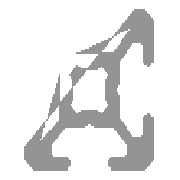
# Autodesk Inventor part: 3 842 992 890-25mm
Saved by Autodesk Inventor 2011 SP1 (Build 150282100, 282)
## iProperties
Created: 2011-02-24
Part Number: 3 842 992 890-25mm
Description: PROFILE 20x20R, -/-
Document SubType Name: Modeling
Designer: SRW
Density: 2.71 g/cm^3
Categories: <MemberInstance><Categories><Category DisplayName="Structural Shapes" InternalName="089c4875-fa83-4c05-b084-43b9cc11f5ed" Mnemonic="GRDR"><CategoryParameter DisplayName="Custom Base Point" InternalName="4f1d1b73-316d-484b-a3df-9cbabb16eb77" Mnemonic="shpBasePoint"/><CategoryParameter DisplayName="FG Authored" InternalName="9c666724-f362-4ea7-ac62-f6a007de5c69" Mnemonic="shpFGAuto"/><CategoryParameter DisplayName="Legacy Member ID" InternalName="340afe4f-75d7-48d3-ab7d-943f3c3da468" Mnemonic="LegacyMemberID"/><CategoryParameter DisplayName="Base Length" InternalName="42e34263-8f20-4d0e-ad48-bf1385b87c24" Mnemonic="shplen"/><CategoryParameter DisplayName="Distance of the Center of Gravity X-X" InternalName="26c9bdb8-9c79-4b4f-a92e-8e197583c9c4" Mnemonic="grcendistX"/><CategoryParameter DisplayName="Distance of the Center of Gravity Y-Y" InternalName="bcc4fb17-7af4-436a-8f8c-d0aa3b0248c5" Mnemonic="grcendistY"/><CategoryParameter DisplayName="Torsional Rigidity Modulus" InternalName="26c1ec35-5026-4c63-ad0a-751cf684a536" Mnemonic="torrigmod"/><CategoryParameter DisplayName="Torsional Section Modulus" InternalName="7c55a8dc-8844-49f9-a867-cc677b30ec9a" Mnemonic="torsecmod"/><CategoryParameter DisplayName="Coefficient of Shear Displacement" InternalName="de4c90c6-aaa8-468f-a335-6737b311b5d3" Mnemonic="shdispc"/><CategoryParameter DisplayName="Section Area" InternalName="1ff91680-64b0-4202-b9a3-7fd3f94bba3b" Mnemonic="secarea"/><CategoryParameter DisplayName="Moment of Inertia (x)" InternalName="4cd780bc-73d7-43ac-917a-579e5cbd684d" Mnemonic="inermomx"/><CategoryParameter DisplayName="Moment of Inertia (y)" InternalName="4b9f58ea-bced-460e-81ea-3d29ca5a49e3" Mnemonic="inermomy"/><CategoryParameter DisplayName="Section Module (x)" InternalName="72cfad18-cf51-4ed4-aaa7-c6b224f8419f" Mnemonic="secmodx"/><CategoryParameter DisplayName="Section Module (y)" InternalName="59eaa5e9-d227-48dc-b6c1-6920f96e0f95" Mnemonic="secmody"/><CategoryParameter DisplayName="Radius of Gyration (x)" InternalName="25778675-03e9-40c1-b6a8-4a9ed693320d" Mnemonic="gyrradx"/><CategoryParameter DisplayName="Radius of Gyration (y)" InternalName="bfa18ebe-1636-4dbe-8d42-b263e0b73184" Mnemonic="gyrrady"/><CategoryParameter DisplayName="Shape Thickness" InternalName="d109cf76-8eb4-42fc-9800-4409734adc67" Mnemonic="shpthick"/><CategoryParameter DisplayName="Second Shape Thickness" InternalName="9251a8e1-85fd-4e47-af99-afdb762317d9" Mnemonic="shpthick2"/><CategoryParameter DisplayName="Shape Width" InternalName="7c717d54-a18f-4666-b4d4-573cce22c62c" Mnemonic="shpwdth"/><CategoryParameter DisplayName="Shape Height" InternalName="50274e7d-5ac0-4796-92cb-c59e54983c67" Mnemonic="shpheig"/><CategoryParameter DisplayName="Mass per Length Unit" InternalName="0bb95a10-148f-4027-a459-38d7b056702a" Mnemonic="shpmass"/><CategoryParameter DisplayName="Section Designation" InternalName="5a64d034-428d-49c8-ba32-7619764de20f" Mnemonic="shpdes"/><Category DisplayName="Other" InternalName="f02205ff-2390-476f-921c-0b3185f88e84" Mnemonic="OTHSHP"><CategoryParameter DisplayName="Moment of Inertia (x)" InternalName="ec6737bc-264f-43ed-b0bd-f6d410c2718d" Mnemonic="inermomx"/><CategoryParameter DisplayName="Moment of Inertia (y)" InternalName="044c654e-f649-48ac-84cc-650a29ae31ca" Mnemonic="inermomy"/><CategoryParameter DisplayName="Section Module (x)" InternalName="cac70804-9d39-43bb-be17-56ea1f39a6c2" Mnemonic="secmodx"/><CategoryParameter DisplayName="Section Module (y)" InternalName="88b8bff9-a616-4028-93d5-ed4f79680d13" Mnemonic="secmody"/><CategoryParameter DisplayName="Section Area" InternalName="c46ecdf8-b6eb-4db9-8b25-30258930c1e3" Mnemonic="secarea"/><CategoryParameter DisplayName="Radius of Gyration (x)" InternalName="ee72c61e-565e-4fd6-b448-66e1e1abcb7e" Mnemonic="gyrradx"/><CategoryParameter DisplayName="Radius of Gyration (y)" InternalName="743e1dfe-1bba-408b-b985-cf752b207386" Mnemonic="gyrrady"/><CategoryParameter DisplayName="Shape Thickness" InternalName="12b1a788-9233-48fd-a933-2df8ff42b15f" Mnemonic="shpthick"/><CategoryParameter DisplayName="Mass per Length Unit" InternalName="2fd289d6-9394-4d2d-97e6-6659d7d4551d" Mnemonic="shpmass"/></Category></Category></Categories><FamilyTemplate Id="20x20R"><FamilyTemplateParameters><FamilyTemplateParameter ObjectType="kUserParameterObject" ValueType="xs:double" Id="1" ObjectReferenceKey="G_L"/><FamilyTemplateParameter ObjectType="kUserParameterObject" ValueType="xs:double" Id="2" ObjectReferenceKey="G_OFFSET_END"/><FamilyTemplateParameter ObjectType="kUserParameterObject" ValueType="xs:double" Id="3" ObjectReferenceKey="G_OFFSET_START"/><FamilyTemplateParameter ObjectType="kUserParameterObject" ValueType="xs:double" Id="4" ObjectReferenceKey="Length"/><FamilyTemplateParameter ObjectType="kPropertyObject" ValueType="xs:string" Id="7" ObjectReferenceKey="{32853F0F-3444-11d1-9E93-0060B03C1CA6}" SubObjectId="52"/><FamilyTemplateParameter ObjectType="kPartComponentDefinitionObject" ValueType="xs:string" Id="8" SubObjectId="Material"/><FamilyTemplateParameter ObjectType="kPropertyObject" ValueType="xs:string" Id="9" ObjectReferenceKey="{32853F0F-3444-11d1-9E93-0060B03C1CA6}" SubObjectId="5"/><FamilyTemplateParameter ObjectType="kPropertyObject" ValueType="xs:string" Id="10" ObjectReferenceKey="{32853F0F-3444-11D1-9E93-0060B03C1CA6}" SubObjectId="55"/><FamilyTemplateParameter ObjectType="kiPartTableColumnObject" ValueType="xs:string" Id="19" ObjectReferenceKey="FILENAME"/><FamilyTemplateParameter ObjectType="kiPartTableColumnObject" ValueType="xs:string" Id="20" ObjectReferenceKey="MEMBER_REVISION"/></FamilyTemplateParameters></FamilyTemplate><CategoryParameterMap><ParamToTemplateMap><ParamToTemplate CategoryParameter="//CategoryParameter[@InternalName='2675968c-4ce5-49e0-a4f5-552d29089031']" TemplateParameter="7"/><ParamToTemplate CategoryParameter="//CategoryParameter[@InternalName='8b46a4cc-9585-4fed-90c3-899f57e09a73']" TemplateParameter="19"/><ParamToTemplate CategoryParameter="//CategoryParameter[@InternalName='42e34263-8f20-4d0e-ad48-bf1385b87c24']" TemplateParameter="4"/><ParamToTemplate CategoryParameter="//CategoryParameter[@InternalName='818a152a-d3c3-49ca-80ee-df7d91421b8e']" TemplateParameter="8"/><ParamToTemplate CategoryParameter="//CategoryParameter[@InternalName='a65d44b9-392f-4f4f-857b-e4b3d54996fe']" TemplateParameter="20"/><ParamToTemplate CategoryParameter="//CategoryParameter[@InternalName='016b6077-bfbe-49bd-92c9-d8d59c39c941']" TemplateParameter="9"/><ParamToTemplate CategoryParameter="//CategoryParameter[@InternalName='9c666724-f362-4ea7-ac62-f6a007de5c69']" ConstantValue="1"/></ParamToTemplateMap></CategoryParameterMap></MemberInstance>
Stock Number: 3 842 992 890
Material: Aluminum-6061
Mass: 11.0537 g
Surface Area: 46.8226 cm^2
Volume: 4.07885 cm^3
Author: SRW
Autodesk Inventor part; units mm, degrees
ref_plane "YZ Plane" through (0, 0, 0) normal (1, 0, 0) x (0, 1, 0)
ref_plane "XZ Plane" through (0, 0, 0) normal (0, 1, 0) x (-1, 0, 0)
ref_plane "XY Plane" through (0, 0, 0) normal (0, 0, 1) x (1, 0, 0)
sketch "20x20R" plane through (0, 0, 0) normal (0, 0, 1) x (1, 0, 0)
  line L0 (187.9019, 38.2996) -> (189.9183, 38.2996)
  arc A0 (187.9019, 38.2996) -> (187.4101, 37.8078) centre (187.9019, 37.8078) ccw
  line L1 (187.4101, 37.0755) -> (187.4101, 37.8078)
  arc A1 (187.4101, 37.0755) -> (187.566, 36.7127) centre (187.9101, 37.0755) ccw
  line L2 (189.8338, 34.5619) -> (187.566, 36.7127)
  arc A2 (189.8338, 34.5619) -> (190.1778, 34.4247) centre (190.1778, 34.9247) ccw
  line L3 (192.4565, 34.4247) -> (190.1778, 34.4247)
  arc A3 (192.5565, 34.3979) -> (192.4565, 34.4247) centre (192.4565, 34.2247) ccw
  line L4 (193.3101, 33.9628) -> (192.5565, 34.3979)
  arc A4 (193.3101, 33.9628) -> (193.5101, 33.9628) centre (193.4101, 34.1361) ccw
  line L5 (194.2637, 34.3979) -> (193.5101, 33.9628)
  arc A5 (194.3637, 34.4247) -> (194.2637, 34.3979) centre (194.3637, 34.2247) ccw
  line L6 (196.6423, 34.4247) -> (194.3637, 34.4247)
  arc A6 (196.6423, 34.4247) -> (196.9864, 34.5619) centre (196.6423, 34.9247) ccw
  arc A7 (191.4101, 25.3593) -> (191.1101, 24.4593) centre (191.4101, 24.8593) ccw
  arc A8 (191.1101, 24.4593) -> (199.5953, 21.3807) centre (200.4101, 36.8593) ccw
  arc A9 (199.5953, 21.3807) -> (199.9751, 22.2336) centre (199.6216, 21.88) ccw
  line L7 (199.9751, 22.2336) -> (196.9959, 25.2128)
  arc A10 (196.9959, 25.2128) -> (196.6423, 25.3593) centre (196.6423, 24.8593) ccw
  line L8 (196.6423, 25.3593) -> (191.4101, 25.3593)
  line L9 (188.9101, 27.8593) -> (188.9101, 33.0915)
  arc A11 (188.9101, 33.0915) -> (188.7636, 33.4451) centre (188.4101, 33.0915) ccw
  line L10 (188.7636, 33.4451) -> (185.7844, 36.4243)
  arc A12 (185.7844, 36.4243) -> (184.9315, 36.0445) centre (185.4308, 36.0708) ccw
  arc A13 (184.9315, 36.0445) -> (188.0101, 27.5593) centre (200.4101, 36.8593) ccw
  arc A14 (188.0101, 27.5593) -> (188.9101, 27.8593) centre (188.4101, 27.8593) ccw
  arc A15 (194.6683, 32.3046) -> (192.1519, 32.3046) centre (193.4101, 29.8593) ccw
  line L11 (192.1519, 32.3046) -> (191.523, 32.807)
  arc A16 (191.523, 32.807) -> (190.4624, 31.7463) centre (193.4101, 29.8593) ccw
  line L12 (190.4624, 31.7463) -> (190.9648, 31.1175)
  arc A17 (190.9648, 31.1175) -> (190.9648, 28.6011) centre (193.4101, 29.8593) ccw
  line L13 (190.9648, 28.6011) -> (190.4624, 27.9722)
  arc A18 (190.4624, 27.9722) -> (191.523, 26.9116) centre (193.4101, 29.8593) ccw
  line L14 (191.523, 26.9116) -> (192.1519, 27.414)
  arc A19 (192.1519, 27.414) -> (194.6683, 27.414) centre (193.4101, 29.8593) ccw
  line L15 (194.6683, 27.414) -> (195.2971, 26.9116)
  arc A20 (195.2971, 26.9116) -> (196.3578, 27.9722) centre (193.4101, 29.8593) ccw
  line L16 (196.3578, 27.9722) -> (195.8554, 28.6011)
  arc A21 (195.8554, 28.6011) -> (195.8554, 31.1175) centre (193.4101, 29.8593) ccw
  line L17 (195.8554, 31.1175) -> (196.3578, 31.7463)
  arc A22 (196.3578, 31.7463) -> (195.2971, 32.807) centre (193.4101, 29.8593) ccw
  line L18 (195.2971, 32.807) -> (194.6683, 32.3046)
  line L19 (199.2541, 36.7127) -> (196.9864, 34.5619)
  arc A23 (199.2541, 36.7127) -> (199.4101, 37.0755) centre (198.9101, 37.0755) ccw
  line L20 (199.4101, 37.8078) -> (199.4101, 37.0755)
  arc A24 (199.4101, 37.8078) -> (198.9183, 38.2996) centre (198.9183, 37.8078) ccw
  line L21 (196.9019, 38.2996) -> (198.9183, 38.2996)
  arc A25 (196.4101, 38.7914) -> (196.9019, 38.2996) centre (196.9019, 38.7914) ccw
  line L22 (196.4101, 39.1093) -> (196.4101, 38.7914)
  arc A26 (196.6101, 39.3093) -> (196.4101, 39.1093) centre (196.6101, 39.1093) ccw
  line L23 (196.7601, 39.3093) -> (196.6101, 39.3093)
  arc A27 (196.7601, 39.3093) -> (196.9601, 39.5093) centre (196.7601, 39.5093) ccw
  line L24 (196.9601, 39.6593) -> (196.9601, 39.5093)
  arc A28 (197.1601, 39.8593) -> (196.9601, 39.6593) centre (197.1601, 39.6593) ccw
  line L25 (201.9101, 39.8593) -> (197.1601, 39.8593)
  arc A29 (203.4101, 38.3593) -> (201.9101, 39.8593) centre (201.9101, 38.3593) ccw
  line L26 (203.4101, 33.6093) -> (203.4101, 38.3593)
  arc A30 (203.2101, 33.4093) -> (203.4101, 33.6093) centre (203.2101, 33.6093) ccw
  line L27 (203.0601, 33.4093) -> (203.2101, 33.4093)
  arc A31 (203.0601, 33.4093) -> (202.8601, 33.2093) centre (203.0601, 33.2093) ccw
  line L28 (202.8601, 33.0593) -> (202.8601, 33.2093)
  arc A32 (202.6601, 32.8593) -> (202.8601, 33.0593) centre (202.6601, 33.0593) ccw
  line L29 (202.2767, 32.8593) -> (202.6601, 32.8593)
  arc A33 (201.7849, 33.3511) -> (202.2767, 32.8593) centre (202.2767, 33.3511) ccw
  line L30 (201.7849, 35.3675) -> (201.7849, 33.3511)
  arc A34 (201.7849, 35.3675) -> (201.2931, 35.8593) centre (201.2931, 35.3675) ccw
  line L31 (200.5609, 35.8593) -> (201.2931, 35.8593)
  arc A35 (200.5609, 35.8593) -> (200.1981, 35.7034) centre (200.5609, 35.3593) ccw
  line L32 (198.0473, 33.4356) -> (200.1981, 35.7034)
  arc A36 (198.0473, 33.4356) -> (197.9101, 33.0915) centre (198.4101, 33.0915) ccw
  line L33 (197.9101, 30.8129) -> (197.9101, 33.0915)
  arc A37 (197.8833, 30.7129) -> (197.9101, 30.8129) centre (197.7101, 30.8129) ccw
  line L34 (197.4482, 29.9593) -> (197.8833, 30.7129)
  arc A38 (197.4482, 29.9593) -> (197.4482, 29.7593) centre (197.6214, 29.8593) ccw
  line L35 (197.8833, 29.0057) -> (197.4482, 29.7593)
  arc A39 (197.9101, 28.9057) -> (197.8833, 29.0057) centre (197.7101, 28.9057) ccw
  line L36 (197.9101, 26.627) -> (197.9101, 28.9057)
  arc A40 (197.9101, 26.627) -> (198.0473, 26.283) centre (198.4101, 26.627) ccw
  line L37 (200.1981, 24.0152) -> (198.0473, 26.283)
  arc A41 (200.1981, 24.0152) -> (200.5609, 23.8593) centre (200.5609, 24.3593) ccw
  line L38 (201.2931, 23.8593) -> (200.5609, 23.8593)
  arc A42 (201.2931, 23.8593) -> (201.7849, 24.3511) centre (201.2931, 24.3511) ccw
  line L39 (201.7849, 26.3675) -> (201.7849, 24.3511)
  arc A43 (202.2767, 26.8593) -> (201.7849, 26.3675) centre (202.2767, 26.3675) ccw
  line L40 (202.6601, 26.8593) -> (202.2767, 26.8593)
  arc A44 (202.8601, 26.6593) -> (202.6601, 26.8593) centre (202.6601, 26.6593) ccw
  line L41 (202.8601, 26.5093) -> (202.8601, 26.6593)
  arc A45 (202.8601, 26.5093) -> (203.0601, 26.3093) centre (203.0601, 26.5093) ccw
  line L42 (203.2101, 26.3093) -> (203.0601, 26.3093)
  arc A46 (203.4101, 26.1093) -> (203.2101, 26.3093) centre (203.2101, 26.1093) ccw
  line L43 (203.4101, 21.3593) -> (203.4101, 26.1093)
  arc A47 (201.9101, 19.8593) -> (203.4101, 21.3593) centre (201.9101, 21.3593) ccw
  line L44 (200.4101, 19.8593) -> (201.9101, 19.8593)
  arc A48 (183.4101, 36.8593) -> (200.4101, 19.8593) centre (200.4101, 36.8593) ccw
  line L45 (183.4101, 38.3593) -> (183.4101, 36.8593)
  arc A49 (184.9101, 39.8593) -> (183.4101, 38.3593) centre (184.9101, 38.3593) ccw
  line L46 (189.6601, 39.8593) -> (184.9101, 39.8593)
  arc A50 (189.8601, 39.6593) -> (189.6601, 39.8593) centre (189.6601, 39.6593) ccw
  line L47 (189.8601, 39.5093) -> (189.8601, 39.6593)
  arc A51 (189.8601, 39.5093) -> (190.0601, 39.3093) centre (190.0601, 39.5093) ccw
  line L48 (190.2101, 39.3093) -> (190.0601, 39.3093)
  arc A52 (190.4101, 39.1093) -> (190.2101, 39.3093) centre (190.2101, 39.1093) ccw
  line L49 (190.4101, 38.7914) -> (190.4101, 39.1093)
  arc A53 (189.9183, 38.2996) -> (190.4101, 38.7914) centre (189.9183, 38.7914) ccw
sketch "Sketch1" plane through (0, 0, 0) normal (0, 0, 1) x (1, 0, 0)
  line L0 (8.4403, 5.5082) -> (8.4403, 3.4918)
  arc A0 (8.4403, 5.5082) -> (7.9485, 6) centre (7.9485, 5.5082) ccw
  line L1 (7.2162, 6) -> (7.9485, 6)
  arc A1 (7.2162, 6) -> (6.8535, 5.8441) centre (7.2162, 5.5) ccw
  line L2 (4.7027, 3.5763) -> (6.8535, 5.8441)
  arc A2 (4.7027, 3.5763) -> (4.5654, 3.2322) centre (5.0654, 3.2322) ccw
  line L3 (4.5654, 0.9536) -> (4.5654, 3.2322)
  arc A3 (4.5387, 0.8536) -> (4.5654, 0.9536) centre (4.3654, 0.9536) ccw
  line L4 (4.1036, 0.1) -> (4.5387, 0.8536)
  arc A4 (4.1036, 0.1) -> (4.1036, -0.1) centre (4.2768, 0) ccw
  line L5 (4.5387, -0.8536) -> (4.1036, -0.1)
  arc A5 (4.5654, -0.9536) -> (4.5387, -0.8536) centre (4.3654, -0.9536) ccw
  line L6 (4.5654, -3.2322) -> (4.5654, -0.9536)
  arc A6 (4.5654, -3.2322) -> (4.7027, -3.5763) centre (5.0654, -3.2322) ccw
  arc A7 (-4.5, 2) -> (-5.4, 2.3) centre (-5, 2) ccw
  arc A8 (-5.4, 2.3) -> (-8.4786, -6.1852) centre (7, -7) ccw
  arc A9 (-8.4786, -6.1852) -> (-7.6257, -6.565) centre (-7.9793, -6.2115) ccw
  line L7 (-7.6257, -6.565) -> (-4.6464, -3.5858)
  arc A10 (-4.6464, -3.5858) -> (-4.5, -3.2322) centre (-5, -3.2322) ccw
  line L8 (-4.5, -3.2322) -> (-4.5, 2)
  line L9 (-2, 4.5) -> (3.2322, 4.5)
  arc A11 (3.2322, 4.5) -> (3.5858, 4.6464) centre (3.2322, 5) ccw
  line L10 (3.5858, 4.6464) -> (6.565, 7.6257)
  arc A12 (6.565, 7.6257) -> (6.1852, 8.4786) centre (6.2115, 7.9793) ccw
  arc A13 (6.1852, 8.4786) -> (-2.3, 5.4) centre (7, -7) ccw
  arc A14 (-2.3, 5.4) -> (-2, 4.5) centre (-2, 5) ccw
  arc A15 (2.4453, -1.2582) -> (2.4453, 1.2582) centre (0, 0) ccw
  line L11 (2.4453, 1.2582) -> (2.9477, 1.8871)
  arc A16 (2.9477, 1.8871) -> (1.8871, 2.9477) centre (0, 0) ccw
  line L12 (1.8871, 2.9477) -> (1.2582, 2.4453)
  arc A17 (1.2582, 2.4453) -> (-1.2582, 2.4453) centre (0, 0) ccw
  line L13 (-1.2582, 2.4453) -> (-1.8871, 2.9477)
  arc A18 (-1.8871, 2.9477) -> (-2.9477, 1.8871) centre (0, 0) ccw
  line L14 (-2.9477, 1.8871) -> (-2.4453, 1.2582)
  arc A19 (-2.4453, 1.2582) -> (-2.4453, -1.2582) centre (0, 0) ccw
  line L15 (-2.4453, -1.2582) -> (-2.9477, -1.8871)
  arc A20 (-2.9477, -1.8871) -> (-1.8871, -2.9477) centre (0, 0) ccw
  line L16 (-1.8871, -2.9477) -> (-1.2582, -2.4453)
  arc A21 (-1.2582, -2.4453) -> (1.2582, -2.4453) centre (0, 0) ccw
  line L17 (1.2582, -2.4453) -> (1.8871, -2.9477)
  arc A22 (1.8871, -2.9477) -> (2.9477, -1.8871) centre (0, 0) ccw
  line L18 (2.9477, -1.8871) -> (2.4453, -1.2582)
  line L19 (6.8535, -5.8441) -> (4.7027, -3.5763)
  arc A23 (6.8535, -5.8441) -> (7.2162, -6) centre (7.2162, -5.5) ccw
  line L20 (7.9485, -6) -> (7.2162, -6)
  arc A24 (7.9485, -6) -> (8.4403, -5.5082) centre (7.9485, -5.5082) ccw
  line L21 (8.4403, -3.4918) -> (8.4403, -5.5082)
  arc A25 (8.9321, -3) -> (8.4403, -3.4918) centre (8.9321, -3.4918) ccw
  line L22 (9.25, -3) -> (8.9321, -3)
  arc A26 (9.45, -3.2) -> (9.25, -3) centre (9.25, -3.2) ccw
  line L23 (9.45, -3.35) -> (9.45, -3.2)
  arc A27 (9.45, -3.35) -> (9.65, -3.55) centre (9.65, -3.35) ccw
  line L24 (9.8, -3.55) -> (9.65, -3.55)
  arc A28 (10, -3.75) -> (9.8, -3.55) centre (9.8, -3.75) ccw
  line L25 (10, -8.5) -> (10, -3.75)
  arc A29 (8.5, -10) -> (10, -8.5) centre (8.5, -8.5) ccw
  line L26 (3.75, -10) -> (8.5, -10)
  arc A30 (3.55, -9.8) -> (3.75, -10) centre (3.75, -9.8) ccw
  line L27 (3.55, -9.65) -> (3.55, -9.8)
  arc A31 (3.55, -9.65) -> (3.35, -9.45) centre (3.35, -9.65) ccw
  line L28 (3.2, -9.45) -> (3.35, -9.45)
  arc A32 (3, -9.25) -> (3.2, -9.45) centre (3.2, -9.25) ccw
  line L29 (3, -8.8666) -> (3, -9.25)
  arc A33 (3.4918, -8.3748) -> (3, -8.8666) centre (3.4918, -8.8666) ccw
  line L30 (5.5082, -8.3748) -> (3.4918, -8.3748)
  arc A34 (5.5082, -8.3748) -> (6, -7.883) centre (5.5082, -7.883) ccw
  line L31 (6, -7.1508) -> (6, -7.883)
  arc A35 (6, -7.1508) -> (5.8441, -6.788) centre (5.5, -7.1508) ccw
  line L32 (3.5763, -4.6372) -> (5.8441, -6.788)
  arc A36 (3.5763, -4.6372) -> (3.2322, -4.5) centre (3.2322, -5) ccw
  line L33 (0.9536, -4.5) -> (3.2322, -4.5)
  arc A37 (0.8536, -4.4732) -> (0.9536, -4.5) centre (0.9536, -4.3) ccw
  line L34 (0.1, -4.0381) -> (0.8536, -4.4732)
  arc A38 (0.1, -4.0381) -> (-0.1, -4.0381) centre (0, -4.2113) ccw
  line L35 (-0.8536, -4.4732) -> (-0.1, -4.0381)
  arc A39 (-0.9536, -4.5) -> (-0.8536, -4.4732) centre (-0.9536, -4.3) ccw
  line L36 (-3.2322, -4.5) -> (-0.9536, -4.5)
  arc A40 (-3.2322, -4.5) -> (-3.5763, -4.6372) centre (-3.2322, -5) ccw
  line L37 (-5.8441, -6.788) -> (-3.5763, -4.6372)
  arc A41 (-5.8441, -6.788) -> (-6, -7.1508) centre (-5.5, -7.1508) ccw
  line L38 (-6, -7.883) -> (-6, -7.1508)
  arc A42 (-6, -7.883) -> (-5.5082, -8.3748) centre (-5.5082, -7.883) ccw
  line L39 (-3.4918, -8.3748) -> (-5.5082, -8.3748)
  arc A43 (-3, -8.8666) -> (-3.4918, -8.3748) centre (-3.4918, -8.8666) ccw
  line L40 (-3, -9.25) -> (-3, -8.8666)
  arc A44 (-3.2, -9.45) -> (-3, -9.25) centre (-3.2, -9.25) ccw
  line L41 (-3.35, -9.45) -> (-3.2, -9.45)
  arc A45 (-3.35, -9.45) -> (-3.55, -9.65) centre (-3.35, -9.65) ccw
  line L42 (-3.55, -9.8) -> (-3.55, -9.65)
  arc A46 (-3.75, -10) -> (-3.55, -9.8) centre (-3.75, -9.8) ccw
  line L43 (-8.5, -10) -> (-3.75, -10)
  arc A47 (-10, -8.5) -> (-8.5, -10) centre (-8.5, -8.5) ccw
  line L44 (-10, -7) -> (-10, -8.5)
  arc A48 (7, 10) -> (-10, -7) centre (7, -7) ccw
  line L45 (8.5, 10) -> (7, 10)
  arc A49 (10, 8.5) -> (8.5, 10) centre (8.5, 8.5) ccw
  line L46 (10, 3.75) -> (10, 8.5)
  arc A50 (9.8, 3.55) -> (10, 3.75) centre (9.8, 3.75) ccw
  line L47 (9.65, 3.55) -> (9.8, 3.55)
  arc A51 (9.65, 3.55) -> (9.45, 3.35) centre (9.65, 3.35) ccw
  line L48 (9.45, 3.2) -> (9.45, 3.35)
  arc A52 (9.25, 3) -> (9.45, 3.2) centre (9.25, 3.2) ccw
  line L49 (8.9321, 3) -> (9.25, 3)
  arc A53 (8.4403, 3.4918) -> (8.9321, 3) centre (8.9321, 3.4918) ccw
  constraints: 1 other
extrude "Extrusion3" add sketch "Sketch1" along normal blind 30
body "Solid2"
